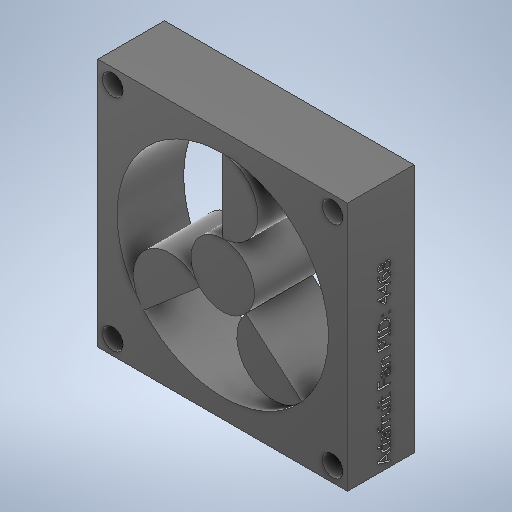
# Autodesk Inventor part: Fan
Saved by Autodesk Inventor 2025 (Build 290162000, 162)
## iProperties
Created: 2025-05-10
Part Number: Fan
Material: Generic
Document SubType Name: Modeling
Designer: thesn
Density: 1 g/cm^3
Appearance: Default
Author: thesn
Autodesk Inventor part; units mm, degrees
ref_plane "YZ Plane" through (0, 0, 0) normal (1, 0, 0) x (0, 1, 0)
ref_plane "XZ Plane" through (0, 0, 0) normal (0, 1, 0) x (-1, 0, 0)
ref_plane "XY Plane" through (0, 0, 0) normal (0, 0, 1) x (1, 0, 0)
sketch "Sketch1" plane through (0, 0, 0) normal (0, 0, 1) x (1, 0, 0)
  line L0 (0, 0) -> (29.99994, 0)
  line L1 (29.99994, 0) -> (29.99994, 29.99994)
  line L2 (29.99994, 29.99994) -> (0, 29.99994)
  line L3 (0, 29.99994) -> (0, 0)
  dimension "d0" = 29.99994
  dimension "d1" = 29.99994
  constraints: 8 end point, 2 parallel, 1 horizontal, 1 perpendicular
  measures "d0" distance of L2.end L1.end
  measures "d1" distance of L1.end L0.end
extrude "Extrusion1" add sketch "Sketch1" along normal blind 8.000009
sketch "Sketch2" plane through (0, 0, 8.000009) normal (0, 0, 1) x (1, 0, 0)
  circle A0 centre (14.99997, 14.99997) radius 12.7
  line L0 (29.99994, 29.99994) -> (0, 29.99994)
  line L1 (0, 29.99994) -> (0, 0)
  point P0 (14.99997, 29.99994)
  point P1 (0, 14.99997)
  dimension "d4" = 0
  dimension "d5" = 0
  dimension "d6" = 25.4
  constraints: 2 midpoint, 1 centre point
  measures "d4" horizontal distance of point (15, 30) A0.centre
  measures "d5" vertical distance of point (0, 15) A0.centre
  measures "d6" diameter of A0
extrude "Extrusion2" cut sketch "Sketch2" against normal blind 8.000009
sketch "Sketch3" plane through (0, 0, 8.000009) normal (0, 0, 1) x (1, 0, 0)
  circle A0 centre (14.99997, 14.99997) radius 3.81
  line L0 (29.99994, 29.99994) -> (0, 29.99994)
  line L1 (0, 29.99994) -> (0, 0)
  line L2 (14.99997, 18.80997) -> (14.99997, 27.69997)
  circle A1 centre (14.99997, 14.99997) radius 12.7
  line L3 (12.232636, 12.381198) -> (5.479746, 6.594297)
  line L4 (17.767304, 12.381198) -> (24.520194, 6.594297)
  arc A2 (14.99997, 18.80997) -> (14.99997, 27.69997) centre (14.791142, 23.25497) ccw
  arc A3 (17.767304, 12.381198) -> (24.520194, 6.594297) centre (21.143749, 9.487748) ccw
  arc A4 (12.232636, 12.381198) -> (5.479746, 6.594297) centre (8.698227, 9.67208) ccw
  point P0 (14.99997, 29.99994)
  point P1 (0, 14.99997)
  point P2 (24.385081, 6.443703)
  point P3 (11.95743, 12.706709)
  point P4 (5.128037, 7.010293)
  dimension "d9" = 7.62
  dimension "d10" = 0
  dimension "d11" = 0
  constraints: 12 point on circle, 6 end point, 4 centre point, 2 midpoint, 1 vertical
  measures "d9" diameter of A0
  measures "d10" horizontal distance of point (15, 30) A0.centre
  measures "d11" vertical distance of point (0, 15) A0.centre
sketch "Sketch3 outline for Extrusion3" plane through (0, 0, 8.000009) normal (0, 0, 1) x (1, 0, 0)
  arc A0 (17.767304, 12.381198) -> (24.385081, 6.443703) centre (21.143749, 9.487748) ccw
  line L0 (24.520194, 6.594297) -> (17.767304, 12.381198)
  arc A1 (24.385081, 6.443703) -> (24.520194, 6.594297) centre (14.99997, 14.99997) ccw
  arc A2 (14.99997, 18.80997) -> (14.99997, 27.69997) centre (14.791142, 23.25497) ccw
  line L1 (14.99997, 27.69997) -> (14.99997, 18.80997)
  arc A3 (11.95743, 12.706709) -> (5.128037, 7.010293) centre (8.698227, 9.67208) ccw
  arc A4 (12.232636, 12.381198) -> (11.95743, 12.706709) centre (14.99997, 14.99997) cw
  line L2 (5.479746, 6.594297) -> (12.232636, 12.381198)
  arc A5 (5.128037, 7.010293) -> (5.479746, 6.594297) centre (14.99997, 14.99997) ccw
  arc A6 (11.95743, 12.706709) -> (12.232636, 12.381198) centre (8.698227, 9.67208) cw
  arc A7 (12.232636, 12.381198) -> (17.767304, 12.381198) centre (14.99997, 14.99997) ccw
  arc A8 (17.767304, 12.381198) -> (14.99997, 18.80997) centre (14.99997, 14.99997) ccw
  arc A9 (14.99997, 18.80997) -> (11.95743, 12.706709) centre (14.99997, 14.99997) ccw
extrude "Extrusion3" add sketch "Sketch3 outline for Extrusion3" against normal blind 8.000009 contours L0 A1 A0 | L1 A2 | A7 A6 A9 A8 | L2 A5 A3 A4
sketch "Sketch4" plane through (0, 0, 8.000009) normal (0, 0, 1) x (1, 0, 0)
  circle A0 centre (1.778, 28.22194) radius 1.25
  line L0 (0, 29.99994) -> (0, 0)
  line L1 (29.99994, 29.99994) -> (0, 29.99994)
  circle A1 centre (28.22194, 28.22194) radius 1.25
  circle A2 centre (28.22194, 1.778) radius 1.25
  circle A3 centre (1.778, 1.778) radius 1.25
  line L2 (0, 0) -> (29.99994, 0)
  line L3 (29.99994, 0) -> (29.99994, 29.99994)
  dimension "d14" = 2.5
  dimension "d15" = 1.778
  dimension "d16" = 1.778
  dimension "d17" = 2.5
  dimension "d18" = 2.5
  dimension "d19" = 2.5
  dimension "d20" = 1.778
  dimension "d21" = 1.778
  dimension "d22" = 1.778
  dimension "d23" = 1.778
  dimension "d24" = 1.778
  dimension "d25" = 1.778
  constraints: 4 centre point
  measures "d14" diameter of A0
  measures "d15" distance from line of L0 A0.centre
  measures "d16" distance from line of L1 A0.centre
  measures "d17" diameter of A1
  measures "d18" diameter of A2
  measures "d19" diameter of A3
  measures "d20" distance from line of L0 A3.centre
  measures "d21" distance from line of L2 A3.centre
  measures "d22" distance from line of L2 A2.centre
  measures "d23" distance from line of L3 A2.centre
  measures "d24" distance from line of L3 A1.centre
  measures "d25" distance from line of L1 A1.centre
extrude "Extrusion4" cut sketch "Sketch4" against normal blind 8.000009 contours A0 | A1 | A2 | A3
sketch "Sketch5" plane through (29.99994, 0, 0) normal (1, 0, 0) x (0, 0, -1)
  line L0 (-4.410246, 0.490027) -> (-4.410246, 43.065697) construction
  line L1 (-4.410246, 43.065697) -> (-1.137474, 43.065697) construction
  line L2 (-1.137474, 43.065697) -> (-1.137474, 0.490027) construction
  line L3 (-1.137474, 0.490027) -> (-4.410246, 0.490027) construction
  line L4 (-2.80844, 0.480147) -> (-4.33244, 0.993911)
  line L5 (-4.33244, 0.993911) -> (-4.33244, 1.243382)
  line L6 (-4.33244, 1.243382) -> (-2.80844, 1.757146)
  line L7 (-2.80844, 1.757146) -> (-2.80844, 1.543489)
  line L8 (-2.80844, 1.543489) -> (-3.234518, 1.405168)
  line L9 (-3.234518, 1.405168) -> (-3.234518, 0.823479)
  line L10 (-3.234518, 0.823479) -> (-2.80844, 0.685159)
  line L11 (-2.80844, 0.685159) -> (-2.80844, 0.480147)
  line L12 (-3.407419, 1.349593) -> (-4.124959, 1.113706)
  line L13 (-4.124959, 1.113706) -> (-3.407419, 0.879055)
  line L14 (-3.407419, 0.879055) -> (-3.407419, 1.349593)
  line L15 (-2.80844, 2.766147) -> (-2.80844, 2.573486)
  line L16 (-2.80844, 2.573486) -> (-2.924531, 2.573486)
  spline S0 degree 2 poles (-2.924531, 2.573486) (-2.887481, 2.529026) (-2.83808, 2.46357) (-2.817085, 2.41911) knots 0 0 0 1 2 2 2
  spline S1 degree 2 poles (-2.817085, 2.41911) (-2.797325, 2.378355) (-2.77633, 2.290669) (-2.77633, 2.232624) knots 0 0 0 1 2 2 2
  spline S2 degree 2 poles (-2.77633, 2.232624) (-2.77633, 2.138763) (-2.854135, 1.980682) (-2.929471, 1.925107) knots 0 0 0 1 2 2 2
  spline S3 degree 2 poles (-2.929471, 1.925107) (-3.004806, 1.869531) (-3.227108, 1.807781) (-3.371604, 1.807781) knots 0 0 0 1 2 2 2
  spline S4 degree 2 poles (-3.371604, 1.807781) (-3.522275, 1.807781) (-3.742106, 1.885586) (-3.824852, 1.953512) knots 0 0 0 1 2 2 2
  spline S5 degree 2 poles (-3.824852, 1.953512) (-3.898952, 2.016497) (-3.984168, 2.193103) (-3.984168, 2.290669) knots 0 0 0 1 2 2 2
  spline S6 degree 2 poles (-3.984168, 2.290669) (-3.984168, 2.375885) (-3.945883, 2.503091) (-3.906362, 2.573486) knots 0 0 0 1 2 2 2
  line L17 (-3.906362, 2.573486) -> (-4.400366, 2.573486)
  line L18 (-4.400366, 2.573486) -> (-4.400366, 2.766147)
  line L19 (-4.400366, 2.766147) -> (-2.80844, 2.766147)
  line L20 (-3.086317, 2.573486) -> (-3.747046, 2.573486)
  spline S7 degree 2 poles (-3.747046, 2.573486) (-3.781627, 2.501855) (-3.807562, 2.388235) (-3.807562, 2.322779) knots 0 0 0 1 2 2 2
  spline S8 degree 2 poles (-3.807562, 2.322779) (-3.807562, 2.174578) (-3.58526, 2.006617) (-3.375309, 2.006617) knots 0 0 0 1 2 2 2
  spline S9 degree 2 poles (-3.375309, 2.006617) (-3.172768, 2.006617) (-2.959111, 2.135058) (-2.959111, 2.277084) knots 0 0 0 1 2 2 2
  spline S10 degree 2 poles (-2.959111, 2.277084) (-2.959111, 2.35242) (-3.028272, 2.505561) (-3.086317, 2.573486) knots 0 0 0 1 2 2 2
  spline S11 degree 2 poles (-2.929471, 3.682523) (-2.912181, 3.659058) (-2.85043, 3.580018) (-2.831905, 3.542967) knots 0 0 0 1 2 2 2
  spline S12 degree 2 poles (-2.831905, 3.542967) (-2.804735, 3.492332) (-2.77633, 3.397236) (-2.77633, 3.310786) knots 0 0 0 1 2 2 2
  spline S13 degree 2 poles (-2.77633, 3.310786) (-2.77633, 3.24039) (-2.829435, 3.113185) (-2.877601, 3.065019) knots 0 0 0 1 2 2 2
  spline S14 degree 2 poles (-2.877601, 3.065019) (-2.924531, 3.019324) (-3.062852, 2.963749) (-3.139422, 2.963749) knots 0 0 0 1 2 2 2
  spline S15 degree 2 poles (-3.139422, 2.963749) (-3.257983, 2.963749) (-3.425944, 3.063784) (-3.474109, 3.172465) knots 0 0 0 1 2 2 2
  spline S16 degree 2 poles (-3.474109, 3.172465) (-3.51857, 3.268796) (-3.551915, 3.530617) (-3.56056, 3.682523) knots 0 0 0 1 2 2 2
  line L21 (-3.56056, 3.682523) -> (-3.59761, 3.682523)
  spline S17 degree 2 poles (-3.59761, 3.682523) (-3.664301, 3.682523) (-3.747046, 3.641768) (-3.770511, 3.604718) knots 0 0 0 1 2 2 2
  spline S18 degree 2 poles (-3.770511, 3.604718) (-3.793977, 3.567668) (-3.808797, 3.461457) (-3.808797, 3.404646) knots 0 0 0 1 2 2 2
  spline S19 degree 2 poles (-3.808797, 3.404646) (-3.808797, 3.337956) (-3.769276, 3.157645) (-3.730991, 3.067489) knots 0 0 0 1 2 2 2
  line L22 (-3.730991, 3.067489) -> (-3.730991, 3.056374)
  line L23 (-3.730991, 3.056374) -> (-3.927357, 3.056374)
  spline S20 degree 2 poles (-3.927357, 3.056374) (-3.942178, 3.109479) (-3.979228, 3.308316) (-3.979228, 3.405881) knots 0 0 0 1 2 2 2
  spline S21 degree 2 poles (-3.979228, 3.405881) (-3.979228, 3.524442) (-3.942178, 3.686228) (-3.894012, 3.750449) knots 0 0 0 1 2 2 2
  spline S22 degree 2 poles (-3.894012, 3.750449) (-3.847082, 3.813434) (-3.697646, 3.875185) (-3.5902, 3.875185) knots 0 0 0 1 2 2 2
  line L24 (-3.5902, 3.875185) -> (-2.80844, 3.875185)
  line L25 (-2.80844, 3.875185) -> (-2.80844, 3.682523)
  line L26 (-2.80844, 3.682523) -> (-2.929471, 3.682523)
  line L27 (-3.090022, 3.682523) -> (-3.407419, 3.682523)
  spline S23 degree 2 poles (-3.407419, 3.682523) (-3.401244, 3.613363) (-3.380249, 3.404646) (-3.360489, 3.339191) knots 0 0 0 1 2 2 2
  spline S24 degree 2 poles (-3.360489, 3.339191) (-3.337024, 3.26262) (-3.239458, 3.162585) (-3.153007, 3.162585) knots 0 0 0 1 2 2 2
  spline S25 degree 2 poles (-3.153007, 3.162585) (-3.054207, 3.162585) (-2.954171, 3.273736) (-2.954171, 3.379946) knots 0 0 0 1 2 2 2
  spline S26 degree 2 poles (-2.954171, 3.379946) (-2.954171, 3.470102) (-3.031977, 3.618303) (-3.090022, 3.682523) knots 0 0 0 1 2 2 2
  line L28 (-4.215114, 4.7471) -> (-4.215114, 4.73722)
  spline S27 degree 2 poles (-4.215114, 4.73722) (-4.224994, 4.711285) (-4.242285, 4.614954) (-4.242285, 4.576669) knots 0 0 0 1 2 2 2
  spline S28 degree 2 poles (-4.242285, 4.576669) (-4.242285, 4.455638) (-4.133604, 4.351898) (-3.990343, 4.351898) knots 0 0 0 1 2 2 2
  line L29 (-3.990343, 4.351898) -> (-3.952058, 4.351898)
  line L30 (-3.952058, 4.351898) -> (-3.952058, 4.67053)
  line L31 (-3.952058, 4.67053) -> (-3.792742, 4.67053)
  line L32 (-3.792742, 4.67053) -> (-3.792742, 4.358073)
  line L33 (-3.792742, 4.358073) -> (-2.80844, 4.358073)
  line L34 (-2.80844, 4.358073) -> (-2.80844, 4.165411)
  line L35 (-2.80844, 4.165411) -> (-3.792742, 4.165411)
  line L36 (-3.792742, 4.165411) -> (-3.792742, 4.035736)
  line L37 (-3.792742, 4.035736) -> (-3.952058, 4.035736)
  line L38 (-3.952058, 4.035736) -> (-3.952058, 4.165411)
  line L39 (-3.952058, 4.165411) -> (-3.990343, 4.165411)
  spline S29 degree 2 poles (-3.990343, 4.165411) (-4.195354, 4.165411) (-4.410246, 4.364248) (-4.410246, 4.549499) knots 0 0 0 1 2 2 2
  spline S30 degree 2 poles (-4.410246, 4.549499) (-4.410246, 4.602604) (-4.399131, 4.70511) (-4.391721, 4.7471) knots 0 0 0 1 2 2 2
  line L40 (-4.391721, 4.7471) -> (-4.215114, 4.7471)
  line L41 (-3.745811, 5.418945) -> (-3.745811, 5.409065)
  spline S31 degree 2 poles (-3.745811, 5.409065) (-3.751986, 5.386834) (-3.754456, 5.338669) (-3.754456, 5.305324) knots 0 0 0 1 2 2 2
  spline S32 degree 2 poles (-3.754456, 5.305324) (-3.754456, 5.227518) (-3.686531, 5.074377) (-3.61984, 5.005217) knots 0 0 0 1 2 2 2
  line L42 (-3.61984, 5.005217) -> (-2.80844, 5.005217)
  line L43 (-2.80844, 5.005217) -> (-2.80844, 4.812556)
  line L44 (-2.80844, 4.812556) -> (-3.952058, 4.812556)
  line L45 (-3.952058, 4.812556) -> (-3.952058, 5.005217)
  line L46 (-3.952058, 5.005217) -> (-3.781627, 5.005217)
  spline S33 degree 2 poles (-3.781627, 5.005217) (-3.875487, 5.110193) (-3.952058, 5.267039) (-3.952058, 5.341139) knots 0 0 0 1 2 2 2
  spline S34 degree 2 poles (-3.952058, 5.341139) (-3.952058, 5.370779) (-3.949588, 5.40042) (-3.945883, 5.418945) knots 0 0 0 1 2 2 2
  line L47 (-3.945883, 5.418945) -> (-3.745811, 5.418945)
  line L48 (-2.80844, 6.457586) -> (-2.80844, 6.264925)
  line L49 (-2.80844, 6.264925) -> (-2.934411, 6.264925)
  spline S35 degree 2 poles (-2.934411, 6.264925) (-2.856605, 6.176005) (-2.77633, 6.016689) (-2.77633, 5.917888) knots 0 0 0 1 2 2 2
  spline S36 degree 2 poles (-2.77633, 5.917888) (-2.77633, 5.843787) (-2.82573, 5.711642) (-2.878836, 5.663476) knots 0 0 0 1 2 2 2
  spline S37 degree 2 poles (-2.878836, 5.663476) (-2.931941, 5.614076) (-3.093727, 5.559736) (-3.209818, 5.559736) knots 0 0 0 1 2 2 2
  line L50 (-3.209818, 5.559736) -> (-3.952058, 5.559736)
  line L51 (-3.952058, 5.559736) -> (-3.952058, 5.752397)
  line L52 (-3.952058, 5.752397) -> (-3.299973, 5.752397)
  spline S38 degree 2 poles (-3.299973, 5.752397) (-3.208583, 5.752397) (-3.088787, 5.765982) (-3.044327, 5.789447) knots 0 0 0 1 2 2 2
  spline S39 degree 2 poles (-3.044327, 5.789447) (-2.999866, 5.812912) (-2.959111, 5.893188) (-2.959111, 5.968523) knots 0 0 0 1 2 2 2
  spline S40 degree 2 poles (-2.959111, 5.968523) (-2.959111, 6.038919) (-3.039387, 6.198235) (-3.097432, 6.264925) knots 0 0 0 1 2 2 2
  line L53 (-3.097432, 6.264925) -> (-3.952058, 6.264925)
  line L54 (-3.952058, 6.264925) -> (-3.952058, 6.457586)
  line L55 (-3.952058, 6.457586) -> (-2.80844, 6.457586)
  line L56 (-2.80844, 6.933065) -> (-2.80844, 6.740403)
  line L57 (-2.80844, 6.740403) -> (-3.952058, 6.740403)
  line L58 (-3.952058, 6.740403) -> (-3.952058, 6.933065)
  line L59 (-3.952058, 6.933065) -> (-2.80844, 6.933065)
  line L60 (-4.142249, 6.94665) -> (-4.142249, 6.728053)
  line L61 (-4.142249, 6.728053) -> (-4.34232, 6.728053)
  line L62 (-4.34232, 6.728053) -> (-4.34232, 6.94665)
  line L63 (-4.34232, 6.94665) -> (-4.142249, 6.94665)
  spline S41 degree 2 poles (-2.78621, 7.561684) (-2.78621, 7.404838) (-2.965286, 7.228232) (-3.159182, 7.228232) knots 0 0 0 1 2 2 2
  line L64 (-3.159182, 7.228232) -> (-3.792742, 7.228232)
  line L65 (-3.792742, 7.228232) -> (-3.792742, 7.098556)
  line L66 (-3.792742, 7.098556) -> (-3.952058, 7.098556)
  line L67 (-3.952058, 7.098556) -> (-3.952058, 7.228232)
  line L68 (-3.952058, 7.228232) -> (-4.28057, 7.228232)
  line L69 (-4.28057, 7.228232) -> (-4.28057, 7.420893)
  line L70 (-4.28057, 7.420893) -> (-3.952058, 7.420893)
  line L71 (-3.952058, 7.420893) -> (-3.952058, 7.77534)
  line L72 (-3.952058, 7.77534) -> (-3.792742, 7.77534)
  line L73 (-3.792742, 7.77534) -> (-3.792742, 7.420893)
  line L74 (-3.792742, 7.420893) -> (-3.248103, 7.420893)
  spline S42 degree 2 poles (-3.248103, 7.420893) (-3.161652, 7.420893) (-3.066557, 7.427068) (-3.025802, 7.448063) knots 0 0 0 1 2 2 2
  spline S43 degree 2 poles (-3.025802, 7.448063) (-2.989986, 7.465353) (-2.954171, 7.543159) (-2.954171, 7.609849) knots 0 0 0 1 2 2 2
  spline S44 degree 2 poles (-2.954171, 7.609849) (-2.954171, 7.656779) (-2.982576, 7.744465) (-2.991221, 7.764225) knots 0 0 0 1 2 2 2
  line L75 (-2.991221, 7.764225) -> (-2.991221, 7.77534)
  line L76 (-2.991221, 7.77534) -> (-2.81832, 7.77534)
  spline S45 degree 2 poles (-2.81832, 7.77534) (-2.8035, 7.721) (-2.78621, 7.609849) (-2.78621, 7.561684) knots 0 0 0 1 2 2 2
  line L77 (-4.152129, 9.498176) -> (-4.152129, 8.789282)
  line L78 (-4.152129, 8.789282) -> (-3.722346, 8.789282)
  line L79 (-3.722346, 8.789282) -> (-3.722346, 9.468536)
  line L80 (-3.722346, 9.468536) -> (-3.542035, 9.468536)
  line L81 (-3.542035, 9.468536) -> (-3.542035, 8.789282)
  line L82 (-3.542035, 8.789282) -> (-2.80844, 8.789282)
  line L83 (-2.80844, 8.789282) -> (-2.80844, 8.58674)
  line L84 (-2.80844, 8.58674) -> (-4.33244, 8.58674)
  line L85 (-4.33244, 8.58674) -> (-4.33244, 9.498176)
  line L86 (-4.33244, 9.498176) -> (-4.152129, 9.498176)
  spline S46 degree 2 poles (-2.929471, 10.302167) (-2.912181, 10.278702) (-2.85043, 10.199661) (-2.831905, 10.162611) knots 0 0 0 1 2 2 2
  spline S47 degree 2 poles (-2.831905, 10.162611) (-2.804735, 10.111976) (-2.77633, 10.01688) (-2.77633, 9.930429) knots 0 0 0 1 2 2 2
  spline S48 degree 2 poles (-2.77633, 9.930429) (-2.77633, 9.860034) (-2.829435, 9.732828) (-2.877601, 9.684663) knots 0 0 0 1 2 2 2
  spline S49 degree 2 poles (-2.877601, 9.684663) (-2.924531, 9.638967) (-3.062852, 9.583392) (-3.139422, 9.583392) knots 0 0 0 1 2 2 2
  spline S50 degree 2 poles (-3.139422, 9.583392) (-3.257983, 9.583392) (-3.425944, 9.683428) (-3.474109, 9.792108) knots 0 0 0 1 2 2 2
  spline S51 degree 2 poles (-3.474109, 9.792108) (-3.51857, 9.888439) (-3.551915, 10.150261) (-3.56056, 10.302167) knots 0 0 0 1 2 2 2
  line L87 (-3.56056, 10.302167) -> (-3.59761, 10.302167)
  spline S52 degree 2 poles (-3.59761, 10.302167) (-3.664301, 10.302167) (-3.747046, 10.261412) (-3.770511, 10.224361) knots 0 0 0 1 2 2 2
  spline S53 degree 2 poles (-3.770511, 10.224361) (-3.793977, 10.187311) (-3.808797, 10.0811) (-3.808797, 10.02429) knots 0 0 0 1 2 2 2
  spline S54 degree 2 poles (-3.808797, 10.02429) (-3.808797, 9.9576) (-3.769276, 9.777288) (-3.730991, 9.687133) knots 0 0 0 1 2 2 2
  line L88 (-3.730991, 9.687133) -> (-3.730991, 9.676018)
  line L89 (-3.730991, 9.676018) -> (-3.927357, 9.676018)
  spline S55 degree 2 poles (-3.927357, 9.676018) (-3.942178, 9.729123) (-3.979228, 9.927959) (-3.979228, 10.025525) knots 0 0 0 1 2 2 2
  spline S56 degree 2 poles (-3.979228, 10.025525) (-3.979228, 10.144086) (-3.942178, 10.305872) (-3.894012, 10.370092) knots 0 0 0 1 2 2 2
  spline S57 degree 2 poles (-3.894012, 10.370092) (-3.847082, 10.433078) (-3.697646, 10.494828) (-3.5902, 10.494828) knots 0 0 0 1 2 2 2
  line L90 (-3.5902, 10.494828) -> (-2.80844, 10.494828)
  line L91 (-2.80844, 10.494828) -> (-2.80844, 10.302167)
  line L92 (-2.80844, 10.302167) -> (-2.929471, 10.302167)
  line L93 (-3.090022, 10.302167) -> (-3.407419, 10.302167)
  spline S58 degree 2 poles (-3.407419, 10.302167) (-3.401244, 10.233006) (-3.380249, 10.02429) (-3.360489, 9.958835) knots 0 0 0 1 2 2 2
  spline S59 degree 2 poles (-3.360489, 9.958835) (-3.337024, 9.882264) (-3.239458, 9.782228) (-3.153007, 9.782228) knots 0 0 0 1 2 2 2
  spline S60 degree 2 poles (-3.153007, 9.782228) (-3.054207, 9.782228) (-2.954171, 9.893379) (-2.954171, 9.99959) knots 0 0 0 1 2 2 2
  spline S61 degree 2 poles (-2.954171, 9.99959) (-2.954171, 10.089745) (-3.031977, 10.237946) (-3.090022, 10.302167) knots 0 0 0 1 2 2 2
  line L94 (-2.80844, 11.663146) -> (-2.80844, 11.470484)
  line L95 (-2.80844, 11.470484) -> (-3.460524, 11.470484)
  spline S62 degree 2 poles (-3.460524, 11.470484) (-3.539565, 11.470484) (-3.675416, 11.455664) (-3.716171, 11.433434) knots 0 0 0 1 2 2 2
  spline S63 degree 2 poles (-3.716171, 11.433434) (-3.759396, 11.409969) (-3.801387, 11.325989) (-3.801387, 11.254358) knots 0 0 0 1 2 2 2
  spline S64 degree 2 poles (-3.801387, 11.254358) (-3.801387, 11.182728) (-3.724816, 11.030822) (-3.663066, 10.957956) knots 0 0 0 1 2 2 2
  line L96 (-3.663066, 10.957956) -> (-2.80844, 10.957956)
  line L97 (-2.80844, 10.957956) -> (-2.80844, 10.765295)
  line L98 (-2.80844, 10.765295) -> (-3.952058, 10.765295)
  line L99 (-3.952058, 10.765295) -> (-3.952058, 10.957956)
  line L100 (-3.952058, 10.957956) -> (-3.824852, 10.957956)
  spline S65 degree 2 poles (-3.824852, 10.957956) (-3.902657, 11.044407) (-3.984168, 11.211133) (-3.984168, 11.304993) knots 0 0 0 1 2 2 2
  spline S66 degree 2 poles (-3.984168, 11.304993) (-3.984168, 11.472954) (-3.761866, 11.663146) (-3.55068, 11.663146) knots 0 0 0 1 2 2 2
  line L101 (-3.55068, 11.663146) -> (-2.80844, 11.663146)
  spline S67 degree 2 poles (-3.873017, 13.566293) (-3.774216, 13.566293) (-3.596375, 13.495898) (-3.534625, 13.432912) knots 0 0 0 1 2 2 2
  spline S68 degree 2 poles (-3.534625, 13.432912) (-3.456819, 13.353872) (-3.376544, 13.140215) (-3.376544, 12.977194) knots 0 0 0 1 2 2 2
  line L102 (-3.376544, 12.977194) -> (-3.376544, 12.805528)
  line L103 (-3.376544, 12.805528) -> (-2.80844, 12.805528)
  line L104 (-2.80844, 12.805528) -> (-2.80844, 12.602987)
  line L105 (-2.80844, 12.602987) -> (-4.33244, 12.602987)
  line L106 (-4.33244, 12.602987) -> (-4.33244, 12.985839)
  spline S69 degree 2 poles (-4.33244, 12.985839) (-4.33244, 13.12169) (-4.28798, 13.311882) (-4.237345, 13.384747) knots 0 0 0 1 2 2 2
  spline S70 degree 2 poles (-4.237345, 13.384747) (-4.179299, 13.469963) (-4.000223, 13.566293) (-3.873017, 13.566293) knots 0 0 0 1 2 2 2
  spline S71 degree 2 poles (-3.866842, 13.355107) (-3.945883, 13.355107) (-4.061973, 13.300766) (-4.099024, 13.245191) knots 0 0 0 1 2 2 2
  spline S72 degree 2 poles (-4.099024, 13.245191) (-4.131134, 13.197026) (-4.157069, 13.068585) (-4.157069, 12.973489) knots 0 0 0 1 2 2 2
  line L107 (-4.157069, 12.973489) -> (-4.157069, 12.805528)
  line L108 (-4.157069, 12.805528) -> (-3.549445, 12.805528)
  line L109 (-3.549445, 12.805528) -> (-3.549445, 12.943849)
  spline S73 degree 2 poles (-3.549445, 12.943849) (-3.549445, 13.06735) (-3.588965, 13.219256) (-3.640836, 13.268656) knots 0 0 0 1 2 2 2
  spline S74 degree 2 poles (-3.640836, 13.268656) (-3.686531, 13.314352) (-3.793977, 13.355107) (-3.866842, 13.355107) knots 0 0 0 1 2 2 2
  line L110 (-2.80844, 14.290008) -> (-2.80844, 13.699674)
  line L111 (-2.80844, 13.699674) -> (-2.964051, 13.699674)
  line L112 (-2.964051, 13.699674) -> (-2.964051, 13.89357)
  line L113 (-2.964051, 13.89357) -> (-4.176829, 13.89357)
  line L114 (-4.176829, 13.89357) -> (-4.176829, 13.699674)
  line L115 (-4.176829, 13.699674) -> (-4.33244, 13.699674)
  line L116 (-4.33244, 13.699674) -> (-4.33244, 14.290008)
  line L117 (-4.33244, 14.290008) -> (-4.176829, 14.290008)
  line L118 (-4.176829, 14.290008) -> (-4.176829, 14.096112)
  line L119 (-4.176829, 14.096112) -> (-2.964051, 14.096112)
  line L120 (-2.964051, 14.096112) -> (-2.964051, 14.290008)
  line L121 (-2.964051, 14.290008) -> (-2.80844, 14.290008)
  spline S75 degree 2 poles (-3.569205, 15.742378) (-3.360489, 15.742378) (-3.024567, 15.573181) (-2.930706, 15.431155) knots 0 0 0 1 2 2 2
  spline S76 degree 2 poles (-2.930706, 15.431155) (-2.85784, 15.315065) (-2.80844, 15.076708) (-2.80844, 14.891457) knots 0 0 0 1 2 2 2
  line L122 (-2.80844, 14.891457) -> (-2.80844, 14.540715)
  line L123 (-2.80844, 14.540715) -> (-4.33244, 14.540715)
  line L124 (-4.33244, 14.540715) -> (-4.33244, 14.887752)
  spline S77 degree 2 poles (-4.33244, 14.887752) (-4.33244, 15.102643) (-4.26822, 15.347175) (-4.211409, 15.433626) knots 0 0 0 1 2 2 2
  spline S78 degree 2 poles (-4.211409, 15.433626) (-4.113844, 15.580591) (-3.791507, 15.742378) (-3.569205, 15.742378) knots 0 0 0 1 2 2 2
  spline S79 degree 2 poles (-3.571675, 15.531191) (-3.747046, 15.531191) (-3.995283, 15.4151) (-4.065678, 15.300245) knots 0 0 0 1 2 2 2
  spline S80 degree 2 poles (-4.065678, 15.300245) (-4.113844, 15.218734) (-4.157069, 15.034718) (-4.157069, 14.897632) knots 0 0 0 1 2 2 2
  line L125 (-4.157069, 14.897632) -> (-4.157069, 14.743256)
  line L126 (-4.157069, 14.743256) -> (-2.983811, 14.743256)
  line L127 (-2.983811, 14.743256) -> (-2.983811, 14.897632)
  spline S81 degree 2 poles (-2.983811, 14.897632) (-2.983811, 15.032248) (-3.027037, 15.236024) (-3.085082, 15.31877) knots 0 0 0 1 2 2 2
  spline S82 degree 2 poles (-3.085082, 15.31877) (-3.156712, 15.42498) (-3.393834, 15.531191) (-3.571675, 15.531191) knots 0 0 0 1 2 2 2
  line L128 (-3.660596, 16.300601) -> (-3.660596, 16.05607)
  line L129 (-3.660596, 16.05607) -> (-3.952058, 16.05607)
  line L130 (-3.952058, 16.05607) -> (-3.952058, 16.300601)
  line L131 (-3.952058, 16.300601) -> (-3.660596, 16.300601)
  line L132 (-2.80844, 16.300601) -> (-2.80844, 16.05607)
  line L133 (-2.80844, 16.05607) -> (-3.099902, 16.05607)
  line L134 (-3.099902, 16.05607) -> (-3.099902, 16.300601)
  line L135 (-3.099902, 16.300601) -> (-2.80844, 16.300601)
  line L136 (-3.332084, 18.295139) -> (-3.332084, 18.113593)
  line L137 (-3.332084, 18.113593) -> (-2.80844, 18.113593)
  line L138 (-2.80844, 18.113593) -> (-2.80844, 17.917227)
  line L139 (-2.80844, 17.917227) -> (-3.332084, 17.917227)
  line L140 (-3.332084, 17.917227) -> (-3.332084, 17.244147)
  line L141 (-3.332084, 17.244147) -> (-3.546975, 17.244147)
  line L142 (-3.546975, 17.244147) -> (-4.33244, 17.925872)
  line L143 (-4.33244, 17.925872) -> (-4.33244, 18.113593)
  line L144 (-4.33244, 18.113593) -> (-3.49634, 18.113593)
  line L145 (-3.49634, 18.113593) -> (-3.49634, 18.295139)
  line L146 (-3.49634, 18.295139) -> (-3.332084, 18.295139)
  line L147 (-3.49634, 17.917227) -> (-4.091614, 17.917227)
  line L148 (-4.091614, 17.917227) -> (-3.49634, 17.404698)
  line L149 (-3.49634, 17.404698) -> (-3.49634, 17.917227)
  line L150 (-3.332084, 19.438757) -> (-3.332084, 19.257211)
  line L151 (-3.332084, 19.257211) -> (-2.80844, 19.257211)
  line L152 (-2.80844, 19.257211) -> (-2.80844, 19.060844)
  line L153 (-2.80844, 19.060844) -> (-3.332084, 19.060844)
  line L154 (-3.332084, 19.060844) -> (-3.332084, 18.387765)
  line L155 (-3.332084, 18.387765) -> (-3.546975, 18.387765)
  line L156 (-3.546975, 18.387765) -> (-4.33244, 19.069489)
  line L157 (-4.33244, 19.069489) -> (-4.33244, 19.257211)
  line L158 (-4.33244, 19.257211) -> (-3.49634, 19.257211)
  line L159 (-3.49634, 19.257211) -> (-3.49634, 19.438757)
  line L160 (-3.49634, 19.438757) -> (-3.332084, 19.438757)
  line L161 (-3.49634, 19.060844) -> (-4.091614, 19.060844)
  line L162 (-4.091614, 19.060844) -> (-3.49634, 18.548316)
  line L163 (-3.49634, 18.548316) -> (-3.49634, 19.060844)
  spline S83 degree 2 poles (-3.302443, 20.565084) (-3.185118, 20.565084) (-2.986281, 20.487279) (-2.919591, 20.421823) knots 0 0 0 1 2 2 2
  spline S84 degree 2 poles (-2.919591, 20.421823) (-2.849195, 20.353898) (-2.77633, 20.183467) (-2.77633, 20.080961) knots 0 0 0 1 2 2 2
  spline S85 degree 2 poles (-2.77633, 20.080961) (-2.77633, 19.978455) (-2.84549, 19.809259) (-2.914651, 19.745039) knots 0 0 0 1 2 2 2
  spline S86 degree 2 poles (-2.914651, 19.745039) (-2.997396, 19.665998) (-3.275273, 19.577078) (-3.477815, 19.577078) knots 0 0 0 1 2 2 2
  spline S87 degree 2 poles (-3.477815, 19.577078) (-3.676651, 19.577078) (-3.996518, 19.658588) (-4.115079, 19.743804) knots 0 0 0 1 2 2 2
  spline S88 degree 2 poles (-4.115079, 19.743804) (-4.231169, 19.826549) (-4.360845, 20.088371) (-4.360845, 20.260037) knots 0 0 0 1 2 2 2
  spline S89 degree 2 poles (-4.360845, 20.260037) (-4.360845, 20.310673) (-4.350965, 20.399593) (-4.33985, 20.432938) knots 0 0 0 1 2 2 2
  line L164 (-4.33985, 20.432938) -> (-4.143484, 20.432938)
  line L165 (-4.143484, 20.432938) -> (-4.143484, 20.424293)
  spline S90 degree 2 poles (-4.143484, 20.424293) (-4.158304, 20.395888) (-4.184239, 20.292147) (-4.184239, 20.232867) knots 0 0 0 1 2 2 2
  spline S91 degree 2 poles (-4.184239, 20.232867) (-4.184239, 20.042676) (-3.927357, 19.809259) (-3.675416, 19.787029) knots 0 0 0 1 2 2 2
  spline S92 degree 2 poles (-3.675416, 19.787029) (-3.726051, 19.859895) (-3.781627, 20.013036) (-3.781627, 20.104426) knots 0 0 0 1 2 2 2
  spline S93 degree 2 poles (-3.781627, 20.104426) (-3.781627, 20.193347) (-3.745811, 20.326728) (-3.691471, 20.399593) knots 0 0 0 1 2 2 2
  spline S94 degree 2 poles (-3.691471, 20.399593) (-3.628486, 20.483574) (-3.433354, 20.565084) (-3.302443, 20.565084) knots 0 0 0 1 2 2 2
  spline S95 degree 2 poles (-3.293798, 20.357603) (-3.387659, 20.357603) (-3.514865, 20.308203) (-3.559325, 20.253862) knots 0 0 0 1 2 2 2
  spline S96 degree 2 poles (-3.559325, 20.253862) (-3.591435, 20.213107) (-3.61243, 20.111836) (-3.61243, 20.058731) knots 0 0 0 1 2 2 2
  spline S97 degree 2 poles (-3.61243, 20.058731) (-3.61243, 19.9871) (-3.569205, 19.852485) (-3.52845, 19.787029) knots 0 0 0 1 2 2 2
  spline S98 degree 2 poles (-3.52845, 19.787029) (-3.50622, 19.785794) (-3.464229, 19.783324) (-3.432119, 19.783324) knots 0 0 0 1 2 2 2
  spline S99 degree 2 poles (-3.432119, 19.783324) (-3.274038, 19.783324) (-3.080142, 19.845075) (-3.029507, 19.892005) knots 0 0 0 1 2 2 2
  spline S100 degree 2 poles (-3.029507, 19.892005) (-2.981341, 19.93523) (-2.943056, 20.029091) (-2.943056, 20.082196) knots 0 0 0 1 2 2 2
  spline S101 degree 2 poles (-2.943056, 20.082196) (-2.943056, 20.205697) (-3.118427, 20.357603) (-3.293798, 20.357603) knots 0 0 0 1 2 2 2
  spline S102 degree 2 poles (-2.77386, 21.206053) (-2.77386, 21.092433) (-2.841785, 20.905946) (-2.904771, 20.840491) knots 0 0 0 1 2 2 2
  spline S103 degree 2 poles (-2.904771, 20.840491) (-2.966521, 20.776271) (-3.134482, 20.70958) (-3.229578, 20.70958) knots 0 0 0 1 2 2 2
  spline S104 degree 2 poles (-3.229578, 20.70958) (-3.353079, 20.70958) (-3.56056, 20.841726) (-3.62231, 20.967697) knots 0 0 0 1 2 2 2
  line L166 (-3.62231, 20.967697) -> (-3.628486, 20.967697)
  spline S105 degree 2 poles (-3.628486, 20.967697) (-3.693941, 20.855311) (-3.849552, 20.74663) (-3.965643, 20.74663) knots 0 0 0 1 2 2 2
  spline S106 degree 2 poles (-3.965643, 20.74663) (-4.137309, 20.74663) (-4.36702, 21.005982) (-4.36702, 21.206053) knots 0 0 0 1 2 2 2
  spline S107 degree 2 poles (-4.36702, 21.206053) (-4.36702, 21.413535) (-4.149659, 21.664241) (-3.979228, 21.664241) knots 0 0 0 1 2 2 2
  spline S108 degree 2 poles (-3.979228, 21.664241) (-3.876722, 21.664241) (-3.676651, 21.544446) (-3.61984, 21.43206) knots 0 0 0 1 2 2 2
  line L167 (-3.61984, 21.43206) -> (-3.613665, 21.43206)
  spline S109 degree 2 poles (-3.613665, 21.43206) (-3.551915, 21.565441) (-3.374074, 21.702527) (-3.233283, 21.702527) knots 0 0 0 1 2 2 2
  spline S110 degree 2 poles (-3.233283, 21.702527) (-3.038152, 21.702527) (-2.77386, 21.418475) (-2.77386, 21.206053) knots 0 0 0 1 2 2 2
  spline S111 degree 2 poles (-3.213523, 21.492575) (-3.307383, 21.492575) (-3.418534, 21.418475) (-3.475344, 21.313499) knots 0 0 0 1 2 2 2
  spline S112 degree 2 poles (-3.475344, 21.313499) (-3.495105, 21.278919) (-3.5408, 21.162828) (-3.57044, 21.089963) knots 0 0 0 1 2 2 2
  spline S113 degree 2 poles (-3.57044, 21.089963) (-3.514865, 21.005982) (-3.349374, 20.915827) (-3.244398, 20.915827) knots 0 0 0 1 2 2 2
  spline S114 degree 2 poles (-3.244398, 20.915827) (-3.106077, 20.915827) (-2.925766, 21.082553) (-2.925766, 21.208523) knots 0 0 0 1 2 2 2
  spline S115 degree 2 poles (-2.925766, 21.208523) (-2.925766, 21.336964) (-3.080142, 21.492575) (-3.213523, 21.492575) knots 0 0 0 1 2 2 2
  spline S116 degree 2 poles (-3.976758, 21.46417) (-4.079263, 21.46417) (-4.216349, 21.327084) (-4.216349, 21.204818) knots 0 0 0 1 2 2 2
  spline S117 degree 2 poles (-4.216349, 21.204818) (-4.216349, 21.093668) (-4.094084, 20.951642) (-3.989108, 20.951642) knots 0 0 0 1 2 2 2
  spline S118 degree 2 poles (-3.989108, 20.951642) (-3.913772, 20.951642) (-3.808797, 21.024507) (-3.766806, 21.097373) knots 0 0 0 1 2 2 2
  spline S119 degree 2 poles (-3.766806, 21.097373) (-3.749516, 21.128248) (-3.689001, 21.259159) (-3.671711, 21.312264) knots 0 0 0 1 2 2 2
  spline S120 degree 2 poles (-3.671711, 21.312264) (-3.739636, 21.401185) (-3.884132, 21.46417) (-3.976758, 21.46417) knots 0 0 0 1 2 2 2
  point P0 (0, 0)
  constraints: 2 other
extrude "Extrusion5" cut sketch "Sketch5" against normal blind 0.508
body "Solid1"
